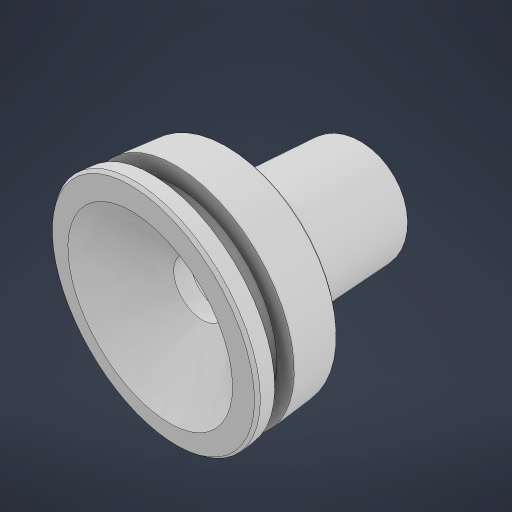
# Autodesk Inventor part: Nozzle
Saved by Autodesk Inventor 2024.1 (Build 281209000, 209)
## iProperties
Created: 2023-02-11
Part Number: Nozzle
Material: Steel
Document SubType Name: Modeling
Designer: Sven
Density: 7.85 g/cm^3
Appearance: Default
Author: Sven
Autodesk Inventor part; units mm, degrees
ref_plane "YZ Plane" through (0, 0, 0) normal (1, 0, 0) x (0, 1, 0)
ref_plane "XZ Plane" through (0, 0, 0) normal (0, 1, 0) x (-1, 0, 0)
ref_plane "XY Plane" through (0, 0, 0) normal (0, 0, 1) x (1, 0, 0)
sketch "Sketch3" plane through (0, 0, 0) normal (0, 1, 0) x (-1, 0, 0)
  line L0 (0, 0) -> (0, 43)
  line L1 (-11, 0) -> (-12, 0)
  line L2 (-12, 0) -> (-12, 28)
  line L3 (-12, 28) -> (-21.75, 28)
  line L4 (-21.75, 28) -> (-21.75, 36.5)
  line L5 (-21.75, 36.5) -> (-18.75, 36.5)
  line L6 (-18.75, 36.5) -> (-18.75, 40)
  line L7 (-18.75, 40) -> (-21.75, 40)
  line L8 (-21.75, 40) -> (-21.75, 43)
  line L9 (-21.75, 43) -> (-17.4, 43)
  line L10 (-17.4, 43) -> (-5.5, 33.0147)
  line L11 (-5.5, 33.0147) -> (-5.5, 29.6753)
  line L12 (-5.5, 29.6753) -> (-11, 0)
  dimension "d1" = 24
  dimension "d2" = 28
  dimension "d3" = 43
  dimension "d5" = 3.5
  dimension "d6" = 43.5
  dimension "d7" = 37.5
  dimension "d8" = 34.8
  dimension "d9" = 11
  dimension "d10" = 29.6753
  dimension "d11" = 9.9853
  dimension "d12" = 22
  dimension "d14" = 10.5
  dimension "d15" = 50
  dimension "d17" = 36.5
  constraints: 26 end point, 6 perpendicular, 3 point on line, 2 horizontal, 2 vertical, 1 parallel
  measures "d1" diameter of L1.end L0
  measures "d2" distance between parallel lines of L3 L1
  measures "d3" distance between parallel lines of L9 L1
  measures "d5" distance between parallel lines of L5 L7
  measures "d6" diameter of L8 L0
  measures "d7" diameter of L6 L0
  measures "d8" diameter of L9.end L0
  measures "d9" diameter of L11 L0
  measures "d10" distance from line of L11.end L1
  measures "d11" distance from line of L10.end L9
  measures "d12" diameter of L1.start L0
  measures "d14" angle of L0 L12
  measures "d15" angle of L0 L10
  measures "d17" distance between parallel lines of L5 L1
revolve "Revolution1" add sketch "Sketch3" angle 360 about axis through (0, 0, 0) along (0, 0, 1)
chamfer "Chamfer1" distance 0.5 angle 45 2 edges at (-21.75, 0, 43) (-21.75, 0, 28)
body "Solid1"
body "Solid2"
